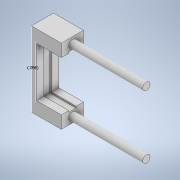
# Autodesk Inventor part: standlower
Saved by Autodesk Inventor 2022 (Build 260153000, 153)
## iProperties
Created: 2022-08-20
Part Number: standlower
Material: Generic
Document SubType Name: Modeling
Designer: yashm
Density: 1 g/cm^3
Appearance: Default
Author: yashm
Autodesk Inventor part; units mm, degrees
ref_plane "YZ Plane" through (0, 0, 0) normal (1, 0, 0) x (0, 1, 0)
ref_plane "XZ Plane" through (0, 0, 0) normal (0, 1, 0) x (-1, 0, 0)
sketch "Sketch1" plane through (0, 0, 0) normal (0, 0, 1) x (1, 0, 0)
  line L0 (0, 0) -> (20.25, 0)
  line L1 (20.25, 0) -> (20.25, 40.5)
  line L2 (20.25, 40.5) -> (0, 40.5)
  line L3 (0, 40.5) -> (0, 0)
  dimension "d0" = 40.5
  dimension "d1" = 20.25
  constraints: 8 end point, 2 parallel, 1 horizontal, 1 perpendicular
  measures "d0" distance of L0.end L1.end
  measures "d1" distance of L1.end L2.end
extrude "Extrusion1" add sketch "Sketch1" along normal blind 15
sketch "Sketch2" plane through (0, 0, 15) normal (0, 0, 1) x (1, 0, 0)
  line L0 (3.5, 37) -> (20.25, 37)
  line L1 (20.25, 37) -> (20.25, 3.5)
  line L2 (20.25, 3.5) -> (3.5, 3.5)
  line L3 (3.5, 3.5) -> (3.5, 37)
  line L4 (20.25, 0) -> (20.25, 40.5) projected
  line L5 (20.25, 40.5) -> (0, 40.5) projected
  line L6 (0, 0) -> (20.25, 0) projected
  dimension "d4" = 16.75
  dimension "d5" = 3.5
  dimension "d6" = 3.5
  constraints: 8 end point, 2 parallel, 1 horizontal, 1 perpendicular, 1 point on line
  measures "d4" distance of L0.start L0.end
  measures "d5" distance between parallel lines of L0 L5
  measures "d6" distance between parallel lines of L6 L2
extrude "Extrusion2" cut sketch "Sketch2" against normal blind 15
ref_plane "Work Plane1" through (0, 0, 7.5) normal (0, 0, 1) x (1, 0, 0)
sketch "Sketch3" plane through (0, 0, 7.5) normal (0, 0, 1) x (1, 0, 0)
  line L0 (2.5, 38) -> (20.25, 38)
  line L1 (20.25, 38) -> (20.25, 2.5)
  line L2 (20.25, 2.5) -> (2.5, 2.5)
  line L3 (2.5, 2.5) -> (2.5, 38)
  line L4 (20.25, 0) -> (20.25, 3.5) projected
  line L5 (20.25, 40.5) -> (0, 40.5) projected
  line L6 (0, 0) -> (20.25, 0) projected
  line L7 (0, 40.5) -> (0, 0) projected
  dimension "d10" = 2.5
  dimension "d11" = 2.5
  dimension "d12" = 2.5
  constraints: 8 end point, 2 parallel, 1 horizontal, 1 perpendicular, 1 point on line
  measures "d10" distance between parallel lines of L5 L0
  measures "d11" distance between parallel lines of L6 L2
  measures "d12" distance between parallel lines of L7 L3
extrude "Extrusion3" cut sketch "Sketch3" along normal mid plane 5
sketch "Sketch4" plane through (20.25, 40.5, 15) normal (1, 0, 0) x (0, 0, -1)
  line L0 (15, 0) -> (0, 0) projected
  line L1 (0, 0) -> (15, 0)
  line L2 (15, 0) -> (15, 5)
  line L3 (15, 5) -> (0, 5)
  line L4 (0, 5) -> (0, 0)
  line L5 (15, -40.5) -> (15, -37) projected
  line L6 (15, -40.5) -> (0, -40.5)
  line L7 (0, -40.5) -> (0, -45.5)
  line L8 (0, -45.5) -> (15, -45.5)
  line L9 (15, -45.5) -> (15, -40.5)
  dimension "d15" = 5
  dimension "d16" = 5
  constraints: 16 end point, 4 parallel, 2 horizontal, 2 perpendicular, 1 point on line
  measures "d15" distance of L1.end L2.end
  measures "d16" distance of L8.end L5.start
extrude "Extrusion4" add sketch "Sketch4" against normal blind 20.25
sketch "Sketch5" plane through (0, 0, 15) normal (0, 0, 1) x (1, 0, 0)
  point P0 (0, 0)
sketch "Sketch6" plane through (20.25, 37, 10) normal (1, 0, 0) x (0, 0, -1)
  circle A0 centre (2.5, 4.5) radius 2.5
  circle A1 centre (2.5, -38) radius 2.5
  line L0 (10, 0) -> (10, 8.5) projected
  line L1 (0, 1) -> (5, 1) projected
  line L2 (10, 8.5) -> (-5, 8.5) projected
  line L3 (5, -34.5) -> (0, -34.5) projected
  point P0 (10, -37)
  dimension "d19" = 7.5
  dimension "d20" = 0
  dimension "d21" = 3.5
  dimension "d22" = 7.5
  dimension "d23" = 3.5
  dimension "d24" = 5
  constraints: 2 centre point, 1 equal radius
  measures "d19" distance from line of L0 A0.centre
  measures "d20" horizontal distance of A1.centre A0.centre
  measures "d21" distance from line of L1 A0.centre
  measures "d22" distance between parallel lines of L2 L1
  measures "d23" distance from line of L3 A1.centre
  measures "d24" diameter of A1
extrude "Extrusion5" add sketch "Sketch6" along normal blind 50
sketch "Sketch7" plane through (0, 0, 15) normal (0, 0, 1) x (1, 0, 0)
  line L0 (0, -5) -> (0, 45.5) projected
  line L1 (2.5, 2.5) -> (2.5, 38) projected
  point P0 (0, 0)
  dimension "d27" = 2.5
  measures "d27" distance between parallel lines of L0 L1
sketch "Sketch8" plane through (0, -5, 0) normal (-1, 0, 0) x (0, 0, 1)
  circle A0 centre (7.5, 25.5) radius 1.5
  line L0 (15, 50.5) -> (0, 50.5) projected
  line L1 (0, 0) -> (15, 0) projected
  line L2 (15, 0) -> (15, 50.5) projected
  line L3 (0, 50.5) -> (0, 0) projected
  point P0 (0, 5)
  dimension "d28" = 50.5
  dimension "d29" = 25
  dimension "d30" = 3
  dimension "d31" = 15
  dimension "d32" = 7.5
  constraints: 1 centre point
  measures "d28" distance between parallel lines of L0 L1
  measures "d29" distance from line of L0 A0.centre
  measures "d30" diameter of A0
  measures "d31" distance between parallel lines of L2 L3
  measures "d32" distance from line of L2 A0.centre
extrude "Extrusion6" add sketch "Sketch8" along normal blind 6 contours A0
body "Solid1"
